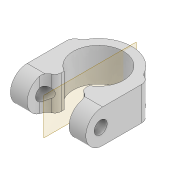
# Autodesk Inventor part: Termination_clip
Saved by Autodesk Inventor 2022 (Build 260153000, 153)
## iProperties
Created: 2022-07-25
Part Number: Termination_clip
Material: Generic
Document SubType Name: Modeling
Designer: dell
Density: 1 g/cm^3
Appearance: Default
Mass: 0.914716 g
Surface Area: 10.3779 cm^2
Volume: 0.914716 cm^3
Author: dell
Autodesk Inventor part; units mm, degrees
ref_plane "XZ Plane" through (0, 0, 0) normal (0, 1, 0) x (-1, 0, 0)
ref_plane "XY Plane" through (0, 0, 0) normal (0, 0, 1) x (1, 0, 0)
sketch "Sketch1" plane through (0, 0, 0) normal (0, 1, 0) x (-1, 0, 0)
  circle A0 centre (0, 0) radius 6
  circle A1 centre (0, 0) radius 8
  line L0 (8, 0) -> (-8, 0)
  line L1 (-8, 0) -> (-8, 12)
  line L2 (-8, 12) -> (8, 12)
  line L3 (8, 12) -> (8, 0)
  line L4 (6, 0) -> (-6, 0)
  line L5 (-6, 0) -> (-6, 12)
  line L6 (-6, 12) -> (6, 12)
  line L7 (6, 12) -> (6, 0)
  line L8 (3, 5.1962) -> (3, 7.4162)
  line L9 (-3, 5.1962) -> (-3, 7.4162)
  line L10 (3, 7.4162) -> (6, 7.4162)
  line L11 (-3, 7.4162) -> (-6, 7.4162)
  line L12 (-11.2, 0) -> (11.2, 0) projected
  dimension "d0" = 12
  dimension "d1" = 2
  dimension "d3" = 4
  dimension "d4" = 3
  dimension "d5" = 3
  constraints: 24 end point, 8 point on circle, 6 point on line, 5 parallel, 3 perpendicular, 2 centre point, 1 coincident, 1 collinear, 1 horizontal, 1 vertical
  measures "d0" diameter of A0
  measures "d1" radial gap between concentric circles of A0 A1
  measures "d3" distance edge to line of A1 L2
  measures "d4" distance between parallel lines of L7 L8
  measures "d5" distance between parallel lines of L5 L9
extrude "Extrusion1" add sketch "Sketch1" along normal blind 8 contours L0 A1 A0 | L7 A1 L0 | A0 L8 A1 L7 | L5 A1 L9 A0 | L0 A1 L5 | A1 L7 L2 L3 | A1 L10 L7 | L1 L2 L5 A1 | L5 L11 A1
fillet "Fillet1" radius 1.5 2 edges at (-3, 4, 7.4162) (3, 4, 7.4162)
sketch "Sketch2" plane through (6, 0, 12) normal (-1, 0, 0) x (0, 0, 1)
  line L0 (0, 0) -> (0, 8) projected
  circle A0 centre (-3.55, 4) radius 1.55
  line L1 (-4.5838, 0) -> (-4.5838, 8) projected
  line L2 (-4.5838, 0) -> (0, 0) projected
  line L3 (-4.5838, 8) -> (0, 8) projected
  point P0 (-12, 0)
  dimension "d9" = 3.1
  dimension "d10" = 2
  dimension "d28" = 4
  constraints: 1 centre point
  measures "d9" diameter of A0
  measures "d10" distance edge to line of A0 L0
  measures "d28" distance from line of L2 A0.centre
extrude "Extrusion2" cut sketch "Sketch2" along normal mid plane 100 contours L1 A0 | A0 L1
sketch "Sketch4" plane through (-8, 0, 0) normal (-1, 0, 0) x (0, 0, 1)
  circle A0 centre (8.45, 4) radius 1.55 projected
  line L0 (0, 0) -> (12, 0) projected
  line L1 (12, 0) -> (12, 8) projected
  line L2 (0, 8) -> (12, 8) projected
  line L3 (0, 0) -> (0, 8) projected
  line L4 (0, 0) -> (0, 0) projected
  line L5 (0, 0) -> (0, 8) projected
  line L6 (0, 8) -> (0, 8) projected
  line L7 (0, 0) -> (0, 8) projected
  line L8 (0, 0) -> (0, 8) projected
  line L9 (0, 8) -> (0, 0)
  line L10 (0, 0) -> (-3, 0)
  line L11 (-3, 0) -> (-3, 8)
  line L12 (-3, 8) -> (0, 8)
  point P0 (0, 0)
  dimension "d22" = 3
  constraints: 8 end point, 3 equal length, 1 perpendicular
  measures "d22" distance between parallel lines of L5 L11
extrude "Extrusion3" add sketch "Sketch4" along normal mid plane 2
fillet "Fillet2" radius 2 2 edges at (-9, 4, -3) (-7.4162, 4, -3)
mirror "Mirror1" about plane through (0, 0, 0) normal (1, 0, 0) of "Extrusion3", "Fillet2"
fillet "Fillet7" radius 4 4 edges at (7.5, 8, 12) (-7.5, 8, 12) (-7.5, 0, 12) (7.5, 0, 12)
thicken "Thicken1" operation add thickness 1 both sides no extend neighbours yes toward (1, 0, 0) faces at (-6, 7.1495, 8.4262)
thicken "Thicken2" operation add thickness 1 both sides no extend neighbours yes toward (-1, 0, 0) faces at (6, 7.1495, 8.4262)
fillet "Fillet8" radius 2 4 edges at (5, 1.4226, 7.4162) (5, 6.5774, 7.4162) (-5, 1.4226, 7.4162) (-5, 6.5774, 7.4162)
body "Solid1"
